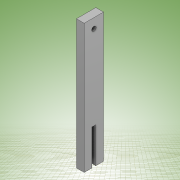
# Autodesk Inventor part: ColumnaSoporte
Saved by Autodesk Inventor 2022 (Build 260153000, 153)
## iProperties
Created: 2022-02-12
Part Number: ColumnaSoporte
Material: Genérico
Document SubType Name: Modeling
Designer: Marco
Density: 1 g/cm^3
Appearance: Valor por defecto
Author: Marco
Autodesk Inventor part; units mm, degrees
ref_plane "YZ Plane" through (0, 0, 0) normal (1, 0, 0) x (0, 1, 0)
ref_plane "XZ Plane" through (0, 0, 0) normal (0, 1, 0) x (-1, 0, 0)
ref_plane "XY Plane" through (0, 0, 0) normal (0, 0, 1) x (1, 0, 0)
sketch "Boceto2" plane through (0, 0, 0) normal (1, 0, 0) x (0, 1, 0)
  line L0 (0, 0) -> (200, 0)
  line L1 (200, 0) -> (200, -30)
  line L2 (200, -30) -> (0, -30)
  circle A0 centre (185, -15) radius 3.5
  line L3 (0, -12) -> (55, -12)
  line L4 (55, -12) -> (55, -18)
  line L5 (55, -18) -> (0, -18)
  line L6 (0, 0) -> (0, -12)
  line L7 (0, -30) -> (0, -18)
  point P0 (200, -15)
  dimension "d2" = 7
  dimension "d3" = 15
  dimension "d7" = 6
  dimension "d8" = 30
  dimension "d9" = 12
  dimension "d10" = 200
  dimension "d11" = 12
  dimension "d12" = 55
  constraints: 16 end point, 2 horizontal, 2 parallel, 2 perpendicular, 2 vertical, 1 centre point, 1 horizontal alignment, 1 midpoint, 1 vertical alignment
  measures "d2" diameter of A0
  measures "d3" horizontal distance of L0.end A0.centre
  measures "d7" distance of L3.end L4.end
  measures "d8" distance of L2.end L0.start
  measures "d9" distance of L0.start L3.start
  measures "d10" distance of L2.end L1.end
  measures "d11" distance of L2.end L5.end
  measures "d12" distance of L3.start L3.end
extrude "Extrusión1" add sketch "Boceto2" along normal blind 12
